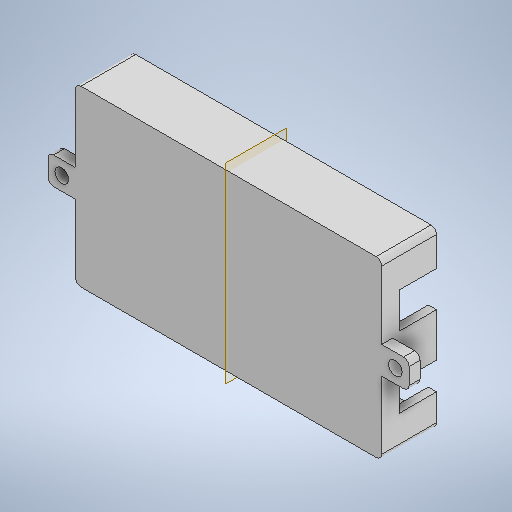
# Autodesk Inventor part: arduino_box
Saved by Autodesk Inventor 2025 (Build 290162000, 162)
## iProperties
Created: 2025-03-03
Part Number: arduino_box
Material: Všeobecné
Document SubType Name: Modeling
Designer: lukas
Density: 1 g/cm^3
Appearance: Výchozí
Author: lukas
## iProperties of the stored document arduino_box_3D tisk.ipt
Created: 2025-03-03
Part Number: arduino_box_3D tisk
Material: Všeobecné
Document SubType Name: Modeling
Designer: lukas
Density: 1 g/cm^3
Appearance: Výchozí
Author: lukas
Autodesk Inventor part; units mm, degrees
(part 1 of 2)
ref_plane "YZ Plane" through (0, 0, 0) normal (1, 0, 0) x (0, 1, 0)
ref_plane "XZ Plane" through (0, 0, 0) normal (0, 1, 0) x (-1, 0, 0)
sketch "Náčrt1" plane through (0, 0, 0) normal (0, 0, 1) x (1, 0, 0)
  line L0 (-99.06, 40.7162) -> (-101.6, 38.1762)
  line L1 (-101.6, 38.1762) -> (-101.6, 3.556)
  line L2 (-101.6, 3.556) -> (-98.044, 0)
  line L3 (-98.044, 0) -> (-1.524, 0)
  line L4 (-1.524, 0) -> (0, 1.524)
  line L5 (0, 1.524) -> (0, 51.8922)
  line L6 (0, 51.8922) -> (-1.524, 53.4162)
  line L7 (-1.524, 53.4162) -> (-97.2966, 53.4162)
  line L8 (-97.2966, 53.4162) -> (-99.06, 51.6528)
  line L9 (-99.06, 51.6528) -> (-99.06, 40.7162)
  circle A0 centre (-89.2556, 50.8762) radius 1.5621
  circle A1 centre (-65.7479, 35.4347) radius 1.3153
  circle A2 centre (-65.7479, 7.4185) radius 1.5621
  circle A3 centre (-96.7486, 2.54) radius 1.5621
  circle A4 centre (-14.1224, 2.54) radius 1.5621
  circle A5 centre (-14.1224, 50.8762) radius 1.5621
  line L10 (-91.7703, 3.1886) -> (-92.8414, 3.1886)
  line L11 (-91.7703, 1.1751) -> (-91.7703, 3.1886)
  line L12 (-92.8414, 1.1751) -> (-91.7703, 1.1751)
  line L13 (-92.8414, 3.1886) -> (-92.8414, 1.1751)
  line L14 (-86.6903, 1.1751) -> (-86.6903, 3.1886)
  line L15 (-87.7614, 1.1751) -> (-86.6903, 1.1751)
  line L16 (-87.7614, 3.1886) -> (-87.7614, 1.1751)
  line L17 (-86.6903, 3.1886) -> (-87.7614, 3.1886)
  line L18 (-81.6103, 1.1751) -> (-81.6103, 3.1886)
  line L19 (-82.6814, 1.1751) -> (-81.6103, 1.1751)
  line L20 (-82.6814, 3.1886) -> (-82.6814, 1.1751)
  line L21 (-81.6103, 3.1886) -> (-82.6814, 3.1886)
  line L22 (-76.5303, 1.1751) -> (-76.5303, 3.1886)
  line L23 (-77.6014, 1.1751) -> (-76.5303, 1.1751)
  line L24 (-77.6014, 3.1886) -> (-77.6014, 1.1751)
  line L25 (-76.5303, 3.1886) -> (-77.6014, 3.1886)
  line L26 (-68.6825, 3.4297) -> (-69.7244, 3.4297)
  line L27 (-68.6825, 1.346) -> (-68.6825, 3.4297)
  line L28 (-69.7244, 1.346) -> (-68.6825, 1.346)
  line L29 (-69.7244, 3.4297) -> (-69.7244, 1.346)
  line L30 (-63.6025, 1.346) -> (-63.6025, 3.4297)
  line L31 (-64.6444, 1.346) -> (-63.6025, 1.346)
  line L32 (-64.6444, 3.4297) -> (-64.6444, 1.346)
  line L33 (-63.6025, 3.4297) -> (-64.6444, 3.4297)
  line L34 (-58.5225, 1.346) -> (-58.5225, 3.4297)
  line L35 (-59.5644, 1.346) -> (-58.5225, 1.346)
  line L36 (-59.5644, 3.4297) -> (-59.5644, 1.346)
  line L37 (-58.5225, 3.4297) -> (-59.5644, 3.4297)
  line L38 (-53.4425, 1.346) -> (-53.4425, 3.4297)
  line L39 (-54.4844, 1.346) -> (-53.4425, 1.346)
  line L40 (-54.4844, 3.4297) -> (-54.4844, 1.346)
  line L41 (-53.4425, 3.4297) -> (-54.4844, 3.4297)
  line L42 (-45.4737, 3.6867) -> (-46.5774, 3.6867)
  line L43 (-45.4737, 1.6118) -> (-45.4737, 3.6867)
  line L44 (-46.5774, 1.6118) -> (-45.4737, 1.6118)
  line L45 (-46.5774, 3.6867) -> (-46.5774, 1.6118)
  line L46 (-40.3937, 1.6118) -> (-40.3937, 3.6867)
  line L47 (-41.4974, 1.6118) -> (-40.3937, 1.6118)
  line L48 (-41.4974, 3.6867) -> (-41.4974, 1.6118)
  line L49 (-40.3937, 3.6867) -> (-41.4974, 3.6867)
  line L50 (-35.3137, 1.6118) -> (-35.3137, 3.6867)
  line L51 (-36.4174, 1.6118) -> (-35.3137, 1.6118)
  line L52 (-36.4174, 3.6867) -> (-36.4174, 1.6118)
  line L53 (-35.3137, 3.6867) -> (-36.4174, 3.6867)
  circle A6 centre (-97.5648, 7.2848) radius 0.5739
  circle A7 centre (-95.0248, 7.2848) radius 0.5739
  circle A8 centre (-95.0248, 9.8248) radius 0.5739
  circle A9 centre (-95.0248, 12.3648) radius 0.5739
  circle A10 centre (-95.0248, 14.9048) radius 0.5739
  circle A11 centre (-95.0248, 17.4448) radius 0.5739
  circle A12 centre (-95.0248, 19.9848) radius 0.5739
  circle A13 centre (-95.0248, 22.5248) radius 0.5739
  circle A14 centre (-95.0248, 25.0648) radius 0.5739
  circle A15 centre (-95.0248, 27.6048) radius 0.5739
  circle A16 centre (-95.0248, 30.1448) radius 0.5739
  circle A17 centre (-95.0248, 32.6848) radius 0.5739
  circle A18 centre (-95.0248, 35.2248) radius 0.5739
  circle A19 centre (-95.0248, 37.7648) radius 0.5739
  circle A20 centre (-95.0248, 40.3048) radius 0.5739
  circle A21 centre (-95.0248, 42.8448) radius 0.5739
  circle A22 centre (-95.0248, 45.3848) radius 0.5739
  circle A23 centre (-95.0248, 47.9248) radius 0.5739
  circle A24 centre (-95.0248, 50.4648) radius 0.5739
  line L54 (-81.8933, 50.0717) -> (-81.8933, 51.6679)
  line L55 (-82.3984, 50.0717) -> (-81.8933, 50.0717)
  line L56 (-82.3984, 51.6679) -> (-82.3984, 50.0717)
  line L57 (-81.8933, 51.6679) -> (-82.3984, 51.6679)
  line L58 (-76.8133, 50.0717) -> (-76.8133, 51.6679)
  line L59 (-77.3184, 50.0717) -> (-76.8133, 50.0717)
  line L60 (-77.3184, 51.6679) -> (-77.3184, 50.0717)
  line L61 (-76.8133, 51.6679) -> (-77.3184, 51.6679)
  line L62 (-71.7333, 50.0717) -> (-71.7333, 51.6679)
  line L63 (-72.2384, 50.0717) -> (-71.7333, 50.0717)
  line L64 (-72.2384, 51.6679) -> (-72.2384, 50.0717)
  line L65 (-71.7333, 51.6679) -> (-72.2384, 51.6679)
  line L66 (-63.4227, 51.9137) -> (-64.2563, 51.9137)
  line L67 (-63.4227, 50.0717) -> (-63.4227, 51.9137)
  line L68 (-64.2563, 50.0717) -> (-63.4227, 50.0717)
  line L69 (-64.2563, 51.9137) -> (-64.2563, 50.0717)
  line L70 (-58.3427, 50.0717) -> (-58.3427, 51.9137)
  line L71 (-59.1763, 50.0717) -> (-58.3427, 50.0717)
  line L72 (-59.1763, 51.9137) -> (-59.1763, 50.0717)
  line L73 (-58.3427, 51.9137) -> (-59.1763, 51.9137)
  line L74 (-53.2627, 50.0717) -> (-53.2627, 51.9137)
  line L75 (-54.0963, 50.0717) -> (-53.2627, 50.0717)
  line L76 (-54.0963, 51.9137) -> (-54.0963, 50.0717)
  line L77 (-53.2627, 51.9137) -> (-54.0963, 51.9137)
  line L78 (-48.1827, 50.0717) -> (-48.1827, 51.9137)
  line L79 (-49.0163, 50.0717) -> (-48.1827, 50.0717)
  line L80 (-49.0163, 51.9137) -> (-49.0163, 50.0717)
  line L81 (-48.1827, 51.9137) -> (-49.0163, 51.9137)
  line L82 (-41.4974, 51.9137) -> (-42.4723, 51.9137)
  line L83 (-41.4974, 50.0717) -> (-41.4974, 51.9137)
  line L84 (-42.4723, 50.0717) -> (-41.4974, 50.0717)
  line L85 (-42.4723, 51.9137) -> (-42.4723, 50.0717)
  line L86 (-36.4174, 50.0717) -> (-36.4174, 51.9137)
  line L87 (-37.3923, 50.0717) -> (-36.4174, 50.0717)
  line L88 (-37.3923, 51.9137) -> (-37.3923, 50.0717)
  line L89 (-36.4174, 51.9137) -> (-37.3923, 51.9137)
  line L90 (-31.3374, 50.0717) -> (-31.3374, 51.9137)
  line L91 (-32.3123, 50.0717) -> (-31.3374, 50.0717)
  line L92 (-32.3123, 51.9137) -> (-32.3123, 50.0717)
  line L93 (-31.3374, 51.9137) -> (-32.3123, 51.9137)
  line L94 (-26.2574, 50.0717) -> (-26.2574, 51.9137)
  line L95 (-27.2323, 50.0717) -> (-26.2574, 50.0717)
  line L96 (-27.2323, 51.9137) -> (-27.2323, 50.0717)
  line L97 (-26.2574, 51.9137) -> (-27.2323, 51.9137)
  circle A25 centre (-20.5945, 47.6784) radius 0.5437
  circle A26 centre (-18.0545, 47.6784) radius 0.5437
  circle A27 centre (-20.5945, 45.1384) radius 0.5437
  circle A28 centre (-15.5145, 45.1384) radius 0.5437
  circle A29 centre (-5.7466, 39.5769) radius 0.4144
  circle A30 centre (-5.7466, 37.0369) radius 0.4144
  line L98 (-7.393, 4.043) -> (-10.0091, 4.043)
  line L99 (-7.393, 3.3305) -> (-7.393, 4.043)
  line L100 (-10.0091, 3.3305) -> (-7.393, 3.3305)
  line L101 (-10.0091, 4.043) -> (-10.0091, 3.3305)
  line L102 (-2.4767, 32.5537) -> (-4.2776, 32.5537)
  line L103 (-2.4767, 31.6979) -> (-2.4767, 32.5537)
  line L104 (-4.2776, 31.6979) -> (-2.4767, 31.6979)
  line L105 (-4.2776, 32.5537) -> (-4.2776, 31.6979)
  line L106 (-2.249, 44.6927) -> (-4.5054, 44.6927)
  line L107 (-2.249, 43.8153) -> (-2.249, 44.6927)
  line L108 (-4.5054, 43.8153) -> (-2.249, 43.8153)
  line L109 (-4.5054, 44.6927) -> (-4.5054, 43.8153)
  line L110 (-5.2737, 10.2292) -> (-5.7128, 10.2292)
  line L111 (-5.2737, 7.3652) -> (-5.2737, 10.2292)
  line L112 (-5.7128, 7.3652) -> (-5.2737, 7.3652)
  line L113 (-5.7128, 10.2292) -> (-5.7128, 7.3652)
  circle A31 centre (-8.2866, 37.0369) radius 0.4144
  line L114 (-11.4599, 10.2292) -> (-12.1472, 10.2292)
  line L115 (-11.4599, 7.3652) -> (-11.4599, 10.2292)
  line L116 (-12.1472, 7.3652) -> (-11.4599, 7.3652)
  line L117 (-12.1472, 10.2292) -> (-12.1472, 7.3652)
  circle A32 centre (-18.0545, 45.1384) radius 0.5437
  circle A33 centre (-15.5145, 47.6784) radius 0.5437
  circle A34 centre (-8.2866, 39.5769) radius 0.4144
  line L118 (-23.7174, 50.0717) -> (-23.7174, 51.9137)
  line L119 (-24.6923, 50.0717) -> (-23.7174, 50.0717)
  line L120 (-24.6923, 51.9137) -> (-24.6923, 50.0717)
  line L121 (-23.7174, 51.9137) -> (-24.6923, 51.9137)
  line L122 (-28.7974, 50.0717) -> (-28.7974, 51.9137)
  line L123 (-29.7723, 50.0717) -> (-28.7974, 50.0717)
  line L124 (-29.7723, 51.9137) -> (-29.7723, 50.0717)
  line L125 (-28.7974, 51.9137) -> (-29.7723, 51.9137)
  line L126 (-33.8774, 50.0717) -> (-33.8774, 51.9137)
  line L127 (-34.8523, 50.0717) -> (-33.8774, 50.0717)
  line L128 (-34.8523, 51.9137) -> (-34.8523, 50.0717)
  line L129 (-33.8774, 51.9137) -> (-34.8523, 51.9137)
  line L130 (-38.9574, 50.0717) -> (-38.9574, 51.9137)
  line L131 (-39.9323, 50.0717) -> (-38.9574, 50.0717)
  line L132 (-39.9323, 51.9137) -> (-39.9323, 50.0717)
  line L133 (-38.9574, 51.9137) -> (-39.9323, 51.9137)
  line L134 (-45.6427, 50.0717) -> (-45.6427, 51.9137)
  line L135 (-46.4763, 50.0717) -> (-45.6427, 50.0717)
  line L136 (-46.4763, 51.9137) -> (-46.4763, 50.0717)
  line L137 (-45.6427, 51.9137) -> (-46.4763, 51.9137)
  line L138 (-50.7227, 50.0717) -> (-50.7227, 51.9137)
  line L139 (-51.5563, 50.0717) -> (-50.7227, 50.0717)
  line L140 (-51.5563, 51.9137) -> (-51.5563, 50.0717)
  line L141 (-50.7227, 51.9137) -> (-51.5563, 51.9137)
  line L142 (-55.8027, 50.0717) -> (-55.8027, 51.9137)
  line L143 (-56.6363, 50.0717) -> (-55.8027, 50.0717)
  line L144 (-56.6363, 51.9137) -> (-56.6363, 50.0717)
  line L145 (-55.8027, 51.9137) -> (-56.6363, 51.9137)
  line L146 (-60.8827, 50.0717) -> (-60.8827, 51.9137)
  line L147 (-61.7163, 50.0717) -> (-60.8827, 50.0717)
  line L148 (-61.7163, 51.9137) -> (-61.7163, 50.0717)
  line L149 (-60.8827, 51.9137) -> (-61.7163, 51.9137)
  line L150 (-69.1933, 50.0717) -> (-69.1933, 51.6679)
  line L151 (-69.6984, 50.0717) -> (-69.1933, 50.0717)
  line L152 (-69.6984, 51.6679) -> (-69.6984, 50.0717)
  line L153 (-69.1933, 51.6679) -> (-69.6984, 51.6679)
  line L154 (-74.2733, 50.0717) -> (-74.2733, 51.6679)
  line L155 (-74.7784, 50.0717) -> (-74.2733, 50.0717)
  line L156 (-74.7784, 51.6679) -> (-74.7784, 50.0717)
  line L157 (-74.2733, 51.6679) -> (-74.7784, 51.6679)
  line L158 (-79.3533, 50.0717) -> (-79.3533, 51.6679)
  line L159 (-79.8584, 50.0717) -> (-79.3533, 50.0717)
  line L160 (-79.8584, 51.6679) -> (-79.8584, 50.0717)
  line L161 (-79.3533, 51.6679) -> (-79.8584, 51.6679)
  line L162 (-84.4333, 50.0717) -> (-84.4333, 51.6679)
  line L163 (-84.9384, 50.0717) -> (-84.4333, 50.0717)
  line L164 (-84.9384, 51.6679) -> (-84.9384, 50.0717)
  line L165 (-84.4333, 51.6679) -> (-84.9384, 51.6679)
  circle A35 centre (-97.5648, 50.4648) radius 0.5739
  circle A36 centre (-97.5648, 47.9248) radius 0.5739
  circle A37 centre (-97.5648, 45.3848) radius 0.5739
  circle A38 centre (-97.5648, 42.8448) radius 0.5739
  circle A39 centre (-97.5648, 40.3048) radius 0.5739
  circle A40 centre (-97.5648, 37.7648) radius 0.5739
  circle A41 centre (-97.5648, 35.2248) radius 0.5739
  circle A42 centre (-97.5648, 32.6848) radius 0.5739
  circle A43 centre (-97.5648, 30.1448) radius 0.5739
  circle A44 centre (-97.5648, 27.6048) radius 0.5739
  circle A45 centre (-97.5648, 25.0648) radius 0.5739
  circle A46 centre (-97.5648, 22.5248) radius 0.5739
  circle A47 centre (-97.5648, 19.9848) radius 0.5739
  circle A48 centre (-97.5648, 17.4448) radius 0.5739
  circle A49 centre (-97.5648, 14.9048) radius 0.5739
  circle A50 centre (-97.5648, 12.3648) radius 0.5739
  circle A51 centre (-97.5648, 9.8248) radius 0.5739
  line L166 (-86.9733, 51.6679) -> (-87.4784, 51.6679)
  line L167 (-86.9733, 50.0717) -> (-86.9733, 51.6679)
  line L168 (-87.4784, 50.0717) -> (-86.9733, 50.0717)
  line L169 (-87.4784, 51.6679) -> (-87.4784, 50.0717)
  line L170 (-32.7737, 1.6118) -> (-32.7737, 3.6867)
  line L171 (-33.8774, 1.6118) -> (-32.7737, 1.6118)
  line L172 (-33.8774, 3.6867) -> (-33.8774, 1.6118)
  line L173 (-32.7737, 3.6867) -> (-33.8774, 3.6867)
  line L174 (-37.8537, 1.6118) -> (-37.8537, 3.6867)
  line L175 (-38.9574, 1.6118) -> (-37.8537, 1.6118)
  line L176 (-38.9574, 3.6867) -> (-38.9574, 1.6118)
  line L177 (-37.8537, 3.6867) -> (-38.9574, 3.6867)
  line L178 (-42.9337, 1.6118) -> (-42.9337, 3.6867)
  line L179 (-44.0374, 1.6118) -> (-42.9337, 1.6118)
  line L180 (-44.0374, 3.6867) -> (-44.0374, 1.6118)
  line L181 (-42.9337, 3.6867) -> (-44.0374, 3.6867)
  line L182 (-50.9025, 1.346) -> (-50.9025, 3.4297)
  line L183 (-51.9444, 1.346) -> (-50.9025, 1.346)
  line L184 (-51.9444, 3.4297) -> (-51.9444, 1.346)
  line L185 (-50.9025, 3.4297) -> (-51.9444, 3.4297)
  line L186 (-55.9825, 1.346) -> (-55.9825, 3.4297)
  line L187 (-57.0244, 1.346) -> (-55.9825, 1.346)
  line L188 (-57.0244, 3.4297) -> (-57.0244, 1.346)
  line L189 (-55.9825, 3.4297) -> (-57.0244, 3.4297)
  line L190 (-61.0625, 1.346) -> (-61.0625, 3.4297)
  line L191 (-62.1044, 1.346) -> (-61.0625, 1.346)
  line L192 (-62.1044, 3.4297) -> (-62.1044, 1.346)
  line L193 (-61.0625, 3.4297) -> (-62.1044, 3.4297)
  line L194 (-66.1425, 1.346) -> (-66.1425, 3.4297)
  line L195 (-67.1844, 1.346) -> (-66.1425, 1.346)
  line L196 (-67.1844, 3.4297) -> (-67.1844, 1.346)
  line L197 (-66.1425, 3.4297) -> (-67.1844, 3.4297)
  line L198 (-73.9903, 1.1751) -> (-73.9903, 3.1886)
  line L199 (-75.0614, 1.1751) -> (-73.9903, 1.1751)
  line L200 (-75.0614, 3.1886) -> (-75.0614, 1.1751)
  line L201 (-73.9903, 3.1886) -> (-75.0614, 3.1886)
  line L202 (-79.0703, 1.1751) -> (-79.0703, 3.1886)
  line L203 (-80.1414, 1.1751) -> (-79.0703, 1.1751)
  line L204 (-80.1414, 3.1886) -> (-80.1414, 1.1751)
  line L205 (-79.0703, 3.1886) -> (-80.1414, 3.1886)
  line L206 (-84.1503, 1.1751) -> (-84.1503, 3.1886)
  line L207 (-85.2214, 1.1751) -> (-84.1503, 1.1751)
  line L208 (-85.2214, 3.1886) -> (-85.2214, 1.1751)
  line L209 (-84.1503, 3.1886) -> (-85.2214, 3.1886)
  line L210 (-89.2303, 1.1751) -> (-89.2303, 3.1886)
  line L211 (-90.3014, 1.1751) -> (-89.2303, 1.1751)
  line L212 (-90.3014, 3.1886) -> (-90.3014, 1.1751)
  line L213 (-89.2303, 3.1886) -> (-90.3014, 3.1886)
  line L214 (0, 64.0994) -> (0, -10.6832)
  line L215 (-121.92, 0) -> (20.32, 0)
  line L216 (0, 0) -> (-101.6, 0)
  line L217 (-101.6, 0) -> (-101.6, 53.4162)
  line L218 (-101.6, 53.4162) -> (0, 53.4162)
  line L219 (0, 53.4162) -> (0, 0)
  dimension "d0" = 0
  constraints: 8 end point, 2 parallel, 1 horizontal, 1 perpendicular, 1 point on line
  measures "d0" distance between parallel lines of L1 L217
extrude "Vysunutí1" add sketch "Náčrt1" along normal blind 2 contours L9 L8 L7 L6 L5 L4 L3 L2 L1 L0 | L0 L217 L218 L8 L9 | L2 L215 L217 | L218 L214 L6 | L4 L214 L215 | A0 | A1 | A2 | A3 | A4 | A5 | L11 L12 L13 L10 | L15 L16 L17 L14 | L19 L20 L21 L18 | L23 L24 L25 L22 | L27 L28 L29 L26 | L31 L32 L33 L30 | L35 L36 L37 L34 | L39 L40 L41 L38 | L43 L44 L45 L42 | L47 L48 L49 L46 | L51 L52 L53 L50 | A6 | A7 | A8 | A9 | A10 | A11 | A12 | A13 | A14 | A15 | A16 | A17 | A18 | A19 | A20 | A21 | A22 | A23 | A24 | L55 L56 L57 L54 | L59 L60 L61 L58 | L63 L64 L65 L62 | L67 L68 L69 L66 | L71 L72 L73 L70 | L75 L76 L77 L74 | L79 L80 L81 L78 | L83 L84 L85 L82 | L87 L88 L89 L86 | L91 L92 L93 L90 | L95 L96 L97 L94 | A25 | A26 | A27 | A28 | A29 | A30 | L99 L100 L101 L98 | L103 L104 L105 L102 | L107 L108 L109 L106 | L111 L112 L113 L110 | A31 | L115 L116 L117 L114 | A32 | A33 | A34 | L119 L120 L121 L118 | L123 L124 L125 L122 | L127 L128 L129 L126 | L131 L132 L133 L130 | L135 L136 L137 L134 | L139 L140 L141 L138 | L143 L144 L145 L142 | L147 L148 L149 L146 | L151 L152 L153 L150 | L155 L156 L157 L154 | L159 L160 L161 L158 | L163 L164 L165 L162 | A35 | A36 | A37 | A38 | A39 | A40 | A41 | A42 | A43 | A44 | A45 | A46 | A47 | A48 | A49 | A50 | A51 | L167 L168 L169 L166 | L171 L172 L173 L170 | L175 L176 L177 L174 | L179 L180 L181 L178 | L183 L184 L185 L182 | L187 L188 L189 L186 | L191 L192 L193 L190 | L195 L196 L197 L194 | L199 L200 L201 L198 | L203 L204 L205 L202 | L207 L208 L209 L206 | L211 L212 L213 L210
sketch "Náčrt2" plane through (0, 0, 0) normal (0, 0, -1) x (-1, 0, 0)
  line L0 (10.795, 12.8905) -> (10.795, 12.2555)
  arc A0 (10.795, 12.2555) -> (10.8585, 12.192) centre (10.8585, 12.2555) ccw
  line L1 (10.8585, 12.192) -> (12.3317, 12.192)
  arc A1 (12.3952, 12.1285) -> (12.3317, 12.192) centre (12.3317, 12.1285) ccw
  line L2 (12.3952, 4.6355) -> (12.3952, 12.1285)
  arc A2 (12.3317, 4.572) -> (12.3952, 4.6355) centre (12.3317, 4.6355) ccw
  line L3 (12.3317, 4.572) -> (10.8585, 4.572)
  arc A3 (10.8585, 4.572) -> (10.795, 4.5085) centre (10.8585, 4.5085) ccw
  line L4 (10.795, 4.5085) -> (10.795, 3.8735)
  arc A4 (10.7315, 3.81) -> (10.795, 3.8735) centre (10.7315, 3.8735) ccw
  line L5 (0, 3.81) -> (10.7315, 3.81)
  line L6 (0, 1.524) -> (0, 3.81)
  line L7 (0, 1.524) -> (1.524, 0)
  line L8 (98.044, 0) -> (1.524, 0)
  line L9 (98.044, 0) -> (101.6, 3.556)
  line L10 (101.6, 38.1762) -> (101.6, 3.556)
  line L11 (99.06, 40.7162) -> (101.6, 38.1762)
  line L12 (99.06, 51.6528) -> (99.06, 40.7162)
  line L13 (97.2966, 53.4162) -> (99.06, 51.6528)
  line L14 (1.524, 53.4162) -> (97.2966, 53.4162)
  line L15 (1.524, 53.4162) -> (0, 51.8922)
  line L16 (0, 44.1452) -> (0, 51.8922)
  line L17 (7.0104, 44.1452) -> (0, 44.1452)
  line L18 (7.0104, 44.2087) -> (7.0104, 44.1452)
  line L19 (9.9568, 44.2087) -> (7.0104, 44.2087)
  line L20 (9.9568, 32.1437) -> (9.9568, 44.2087)
  line L21 (9.9568, 32.1437) -> (7.0104, 32.1437)
  line L22 (7.0104, 32.1437) -> (7.0104, 32.2072)
  line L23 (0, 32.2072) -> (7.0104, 32.2072)
  line L24 (0, 12.954) -> (0, 32.2072)
  line L25 (10.7315, 12.954) -> (0, 12.954)
  arc A5 (10.795, 12.8905) -> (10.7315, 12.954) centre (10.7315, 12.8905) ccw
  line L26 (47.625, 1.3462) -> (47.625, 3.7956)
  line L27 (31.9278, 1.3462) -> (47.625, 1.3462)
  line L28 (31.9278, 3.7956) -> (31.9278, 1.3462)
  line L29 (47.625, 3.7956) -> (31.9278, 3.7956)
  line L30 (21.2598, 49.6824) -> (42.0116, 49.6824)
  line L31 (21.2598, 52.1462) -> (21.2598, 49.6824)
  line L32 (42.0116, 52.1462) -> (21.2598, 52.1462)
  line L33 (42.0116, 49.6824) -> (42.0116, 52.1462)
  line L34 (72.517, 3.81) -> (72.517, 1.3462)
  line L35 (93.345, 3.81) -> (72.517, 3.81)
  line L36 (93.345, 1.3462) -> (93.345, 3.81)
  line L37 (72.517, 1.3462) -> (93.345, 1.3462)
  line L38 (97.536, 5.9182) -> (97.536, 52.197)
  line L39 (92.5576, 5.9182) -> (97.536, 5.9182)
  line L40 (92.5576, 52.197) -> (92.5576, 5.9182)
  line L41 (97.536, 52.197) -> (92.5576, 52.197)
  line L42 (66.7258, 52.1462) -> (66.7258, 49.6824)
  line L43 (87.4776, 52.1462) -> (66.7258, 52.1462)
  line L44 (87.4776, 49.6824) -> (87.4776, 52.1462)
  line L45 (66.7258, 49.6824) -> (87.4776, 49.6824)
  line L46 (43.9928, 49.6824) -> (64.7446, 49.6824)
  line L47 (43.9928, 52.1462) -> (43.9928, 49.6824)
  line L48 (64.7446, 52.1462) -> (43.9928, 52.1462)
  line L49 (64.7446, 49.6824) -> (64.7446, 52.1462)
  line L50 (49.784, 1.3462) -> (70.612, 1.3462)
  line L51 (49.784, 3.81) -> (49.784, 1.3462)
  line L52 (70.612, 3.81) -> (49.784, 3.81)
  line L53 (70.612, 1.3462) -> (70.612, 3.81)
  line L54 (26.4691, 25.5422) -> (26.4691, 24.1341)
  line L55 (29.2341, 25.5422) -> (26.4691, 25.5422)
  line L56 (29.2341, 24.1341) -> (29.2341, 25.5422)
  line L57 (26.4691, 24.1341) -> (29.2341, 24.1341)
  line L58 (6.8597, 20.6667) -> (6.8597, 14.174)
  line L59 (10.1287, 20.6667) -> (6.8597, 20.6667)
  line L60 (10.1287, 14.174) -> (10.1287, 20.6667)
  line L61 (6.8597, 14.174) -> (10.1287, 14.174)
  line L62 (17.0001, 22.4519) -> (17.0001, 19.5908)
  line L63 (19.8206, 22.4519) -> (17.0001, 22.4519)
  line L64 (19.8206, 19.5908) -> (19.8206, 22.4519)
  line L65 (17.0001, 19.5908) -> (19.8206, 19.5908)
  line L66 (20.7541, 17.2167) -> (20.7541, 16.4862)
  line L67 (22.3503, 17.2167) -> (20.7541, 17.2167)
  line L68 (22.3503, 16.4862) -> (22.3503, 17.2167)
  line L69 (20.7541, 16.4862) -> (22.3503, 16.4862)
  line L70 (2.6828, 28.6543) -> (2.6828, 24.1341)
  line L71 (5.8459, 28.6543) -> (2.6828, 28.6543)
  line L72 (5.8459, 24.1341) -> (5.8459, 28.6543)
  line L73 (2.6828, 24.1341) -> (5.8459, 24.1341)
  line L74 (37.9203, 7.1822) -> (37.9203, 6.4561)
  line L75 (39.468, 7.1822) -> (37.9203, 7.1822)
  line L76 (39.468, 6.4561) -> (39.468, 7.1822)
  line L77 (37.9203, 6.4561) -> (39.468, 6.4561)
  line L78 (40.0898, 15.0906) -> (40.0898, 13.6337)
  line L79 (41.0914, 15.0906) -> (40.0898, 15.0906)
  line L80 (41.0914, 13.6337) -> (41.0914, 15.0906)
  line L81 (40.0898, 13.6337) -> (41.0914, 13.6337)
  line L82 (34.709, 15.9464) -> (34.709, 12.6868)
  line L83 (36.5608, 15.9464) -> (34.709, 15.9464)
  line L84 (36.5608, 12.6868) -> (36.5608, 15.9464)
  line L85 (34.709, 12.6868) -> (36.5608, 12.6868)
  line L86 (27.2293, 21.6382) -> (27.2293, 20.877)
  line L87 (28.7931, 21.6382) -> (27.2293, 21.6382)
  line L88 (28.7931, 20.877) -> (28.7931, 21.6382)
  line L89 (27.2293, 20.877) -> (28.7931, 20.877)
  line L90 (11.2848, 29.3883) -> (11.2848, 28.6543)
  line L91 (12.7546, 29.3883) -> (11.2848, 29.3883)
  line L92 (12.7546, 28.6543) -> (12.7546, 29.3883)
  line L93 (11.2848, 28.6543) -> (12.7546, 28.6543)
  line L94 (17.6277, 29.5208) -> (17.6277, 28.6543)
  line L95 (19.2035, 29.5208) -> (17.6277, 29.5208)
  line L96 (19.2035, 28.6543) -> (19.2035, 29.5208)
  line L97 (17.6277, 28.6543) -> (19.2035, 28.6543)
  line L98 (23.859, 29.5208) -> (23.859, 28.6543)
  line L99 (25.4224, 29.5208) -> (23.859, 29.5208)
  line L100 (25.4224, 28.6543) -> (25.4224, 29.5208)
  line L101 (23.859, 28.6543) -> (25.4224, 28.6543)
  line L102 (26.9146, 34.715) -> (26.9146, 33.4422)
  line L103 (28.6926, 34.715) -> (26.9146, 34.715)
  line L104 (28.6926, 33.4422) -> (28.6926, 34.715)
  line L105 (26.9146, 33.4422) -> (28.6926, 33.4422)
  line L106 (27.4303, 40.8048) -> (27.4303, 37.5488)
  line L107 (28.2839, 40.8048) -> (27.4303, 40.8048)
  line L108 (28.2839, 37.5488) -> (28.2839, 40.8048)
  line L109 (27.4303, 37.5488) -> (28.2839, 37.5488)
  line L110 (27.0516, 44.6498) -> (27.0516, 43.8951)
  line L111 (28.4879, 44.6498) -> (27.0516, 44.6498)
  line L112 (28.4879, 43.8951) -> (28.4879, 44.6498)
  line L113 (27.0516, 43.8951) -> (28.4879, 43.8951)
  line L114 (11.1523, 42.3897) -> (11.1523, 41.6172)
  line L115 (12.7546, 42.3897) -> (11.1523, 42.3897)
  line L116 (12.7546, 41.6172) -> (12.7546, 42.3897)
  line L117 (11.1523, 41.6172) -> (12.7546, 41.6172)
  line L118 (11.4503, 38.4446) -> (11.4503, 35.2712)
  line L119 (12.4133, 38.4446) -> (11.4503, 38.4446)
  line L120 (12.4133, 35.2712) -> (12.4133, 38.4446)
  line L121 (11.4503, 35.2712) -> (12.4133, 35.2712)
  line L122 (75.6756, 37.5488) -> (75.6756, 36.1287)
  line L123 (77.4802, 37.5488) -> (75.6756, 37.5488)
  line L124 (77.4802, 36.1287) -> (77.4802, 37.5488)
  line L125 (75.6756, 36.1287) -> (77.4802, 36.1287)
  line L126 (11.8224, 47.7016) -> (11.8224, 44.4497)
  line L127 (13.6426, 47.7016) -> (11.8224, 47.7016)
  line L128 (13.6426, 44.4497) -> (13.6426, 47.7016)
  line L129 (11.8224, 44.4497) -> (13.6426, 44.4497)
  arc A6 (14.5172, 27.5532) -> (14.5172, 23.7943) centre (14.8394, 25.6738) ccw
  line L130 (22.4159, 27.5532) -> (14.5172, 27.5532)
  arc A7 (22.4159, 23.7943) -> (22.4159, 27.5532) centre (22.0937, 25.6738) ccw
  line L131 (14.5172, 23.7943) -> (22.4159, 23.7943)
  circle A8 centre (25.2188, 8.6007) radius 3.302
  line L132 (67.919, 27.2067) -> (67.919, 27.8713)
  line L133 (66.903, 26.1907) -> (67.919, 27.2067)
  line L134 (63.5244, 26.1907) -> (66.903, 26.1907)
  line L135 (62.5084, 27.2067) -> (63.5244, 26.1907)
  line L136 (62.5084, 27.8713) -> (62.5084, 27.2067)
  line L137 (63.5244, 28.8873) -> (62.5084, 27.8713)
  line L138 (66.903, 28.8873) -> (63.5244, 28.8873)
  line L139 (67.919, 27.8713) -> (66.903, 28.8873)
  line L140 (15.9051, 48.775) -> (15.2447, 48.775)
  line L141 (16.9211, 47.759) -> (15.9051, 48.775)
  line L142 (16.9211, 44.3808) -> (16.9211, 47.759)
  line L143 (15.9051, 43.3648) -> (16.9211, 44.3808)
  line L144 (15.2447, 43.3648) -> (15.9051, 43.3648)
  line L145 (14.2287, 44.3808) -> (15.2447, 43.3648)
  line L146 (14.2287, 47.759) -> (14.2287, 44.3808)
  line L147 (15.2447, 48.775) -> (14.2287, 47.759)
  line L148 (20.8327, 48.775) -> (19.8167, 47.759)
  line L149 (21.4931, 48.775) -> (20.8327, 48.775)
  line L150 (22.5091, 47.759) -> (21.4931, 48.775)
  line L151 (22.5091, 44.3808) -> (22.5091, 47.759)
  line L152 (21.4931, 43.3648) -> (22.5091, 44.3808)
  line L153 (20.8327, 43.3648) -> (21.4931, 43.3648)
  line L154 (19.8167, 44.3808) -> (20.8327, 43.3648)
  line L155 (19.8167, 47.759) -> (19.8167, 44.3808)
  circle A9 centre (14.1224, 50.8762) radius 1.5621
  circle A10 centre (14.1224, 2.54) radius 1.5621
  circle A11 centre (96.7486, 2.54) radius 1.5621
  circle A12 centre (65.7479, 7.4185) radius 1.5621
  circle A13 centre (65.7479, 35.4347) radius 1.3153
  circle A14 centre (89.2556, 50.8762) radius 1.5621
  line L156 (18.0387, 48.775) -> (17.0227, 47.759)
  line L157 (18.6991, 48.775) -> (18.0387, 48.775)
  line L158 (19.7151, 47.759) -> (18.6991, 48.775)
  line L159 (19.7151, 44.3808) -> (19.7151, 47.759)
  line L160 (18.6991, 43.3648) -> (19.7151, 44.3808)
  line L161 (18.0387, 43.3648) -> (18.6991, 43.3648)
  line L162 (17.0227, 44.3808) -> (18.0387, 43.3648)
  line L163 (17.0227, 47.759) -> (17.0227, 44.3808)
  line L164 (67.919, 24.4127) -> (67.919, 25.0773)
  line L165 (66.903, 23.3967) -> (67.919, 24.4127)
  line L166 (63.5244, 23.3967) -> (66.903, 23.3967)
  line L167 (62.5084, 24.4127) -> (63.5244, 23.3967)
  line L168 (62.5084, 25.0773) -> (62.5084, 24.4127)
  line L169 (63.5244, 26.0933) -> (62.5084, 25.0773)
  line L170 (66.903, 26.0933) -> (63.5244, 26.0933)
  line L171 (67.919, 25.0773) -> (66.903, 26.0933)
  line L172 (67.919, 30.0007) -> (67.919, 30.6653)
  line L173 (66.903, 28.9847) -> (67.919, 30.0007)
  line L174 (63.5244, 28.9847) -> (66.903, 28.9847)
  line L175 (62.5084, 30.0007) -> (63.5244, 28.9847)
  line L176 (62.5084, 30.6653) -> (62.5084, 30.0007)
  line L177 (63.5244, 31.6813) -> (62.5084, 30.6653)
  line L178 (66.903, 31.6813) -> (63.5244, 31.6813)
  line L179 (67.919, 30.6653) -> (66.903, 31.6813)
  circle A15 centre (18.0299, 8.6007) radius 3.302
  line L180 (71.3142, 30.7771) -> (71.3142, 24.4981)
  line L181 (77.7751, 30.7771) -> (71.3142, 30.7771)
  line L182 (77.7751, 24.4981) -> (77.7751, 30.7771)
  line L183 (71.3142, 24.4981) -> (77.7751, 24.4981)
  line L184 (80.4259, 38.4446) -> (80.4259, 35.0406)
  line L185 (81.6732, 38.4446) -> (80.4259, 38.4446)
  line L186 (81.6732, 35.0406) -> (81.6732, 38.4446)
  line L187 (80.4259, 35.0406) -> (81.6732, 35.0406)
  line L188 (11.1523, 34.5656) -> (11.1523, 33.6296)
  line L189 (12.7546, 34.5656) -> (11.1523, 34.5656)
  line L190 (12.7546, 33.6296) -> (12.7546, 34.5656)
  line L191 (11.1523, 33.6296) -> (12.7546, 33.6296)
  line L192 (11.1523, 40.0722) -> (11.1523, 39.1768)
  line L193 (12.7546, 40.0722) -> (11.1523, 40.0722)
  line L194 (12.7546, 39.1768) -> (12.7546, 40.0722)
  line L195 (11.1523, 39.1768) -> (12.7546, 39.1768)
  line L196 (7.126, 45.5392) -> (7.126, 44.4497)
  line L197 (9.0679, 45.5392) -> (7.126, 45.5392)
  line L198 (9.0679, 44.4497) -> (9.0679, 45.5392)
  line L199 (7.126, 44.4497) -> (9.0679, 44.4497)
  line L200 (26.9146, 42.5941) -> (26.9146, 41.3621)
  line L201 (28.6926, 42.5941) -> (26.9146, 42.5941)
  line L202 (28.6926, 41.3621) -> (28.6926, 42.5941)
  line L203 (26.9146, 41.3621) -> (28.6926, 41.3621)
  line L204 (26.9146, 37.0281) -> (26.9146, 35.7687)
  line L205 (28.6926, 37.0281) -> (26.9146, 37.0281)
  line L206 (28.6926, 35.7687) -> (28.6926, 37.0281)
  line L207 (26.9146, 35.7687) -> (28.6926, 35.7687)
  line L208 (27.4303, 32.4686) -> (27.4303, 29.2498)
  line L209 (28.4879, 32.4686) -> (27.4303, 32.4686)
  line L210 (28.4879, 29.2498) -> (28.4879, 32.4686)
  line L211 (27.4303, 29.2498) -> (28.4879, 29.2498)
  line L212 (20.7541, 29.5208) -> (20.7541, 28.6543)
  line L213 (22.2343, 29.5208) -> (20.7541, 29.5208)
  line L214 (22.2343, 28.6543) -> (22.2343, 29.5208)
  line L215 (20.7541, 28.6543) -> (22.2343, 28.6543)
  line L216 (14.4129, 29.3883) -> (14.4129, 28.6543)
  line L217 (15.946, 29.3883) -> (14.4129, 29.3883)
  line L218 (15.946, 28.6543) -> (15.946, 29.3883)
  line L219 (14.4129, 28.6543) -> (15.946, 28.6543)
  line L220 (11.1523, 31.0171) -> (11.1523, 30.3418)
  line L221 (12.7546, 31.0171) -> (11.1523, 31.0171)
  line L222 (12.7546, 30.3418) -> (12.7546, 31.0171)
  line L223 (11.1523, 30.3418) -> (12.7546, 30.3418)
  line L224 (27.1372, 18.3326) -> (27.1372, 17.5844)
  line L225 (28.6926, 18.3326) -> (27.1372, 18.3326)
  line L226 (28.6926, 17.5844) -> (28.6926, 18.3326)
  line L227 (27.1372, 17.5844) -> (28.6926, 17.5844)
  line L228 (37.7953, 15.9464) -> (37.7953, 12.6868)
  line L229 (39.07, 15.9464) -> (37.7953, 15.9464)
  line L230 (39.07, 12.6868) -> (39.07, 15.9464)
  line L231 (37.7953, 12.6868) -> (39.07, 12.6868)
  line L232 (33.0606, 15.564) -> (33.0606, 13.4334)
  line L233 (34.0257, 15.564) -> (33.0606, 15.564)
  line L234 (34.0257, 13.4334) -> (34.0257, 15.564)
  line L235 (33.0606, 13.4334) -> (34.0257, 13.4334)
  line L236 (8.4942, 26.9002) -> (8.4942, 24.1341)
  line L237 (9.6416, 26.9002) -> (8.4942, 26.9002)
  line L238 (9.6416, 24.1341) -> (9.6416, 26.9002)
  line L239 (8.4942, 24.1341) -> (9.6416, 24.1341)
  line L240 (14.0173, 18.0486) -> (14.0173, 16.4862)
  line L241 (14.8086, 18.0486) -> (14.0173, 18.0486)
  line L242 (14.8086, 16.4862) -> (14.8086, 18.0486)
  line L243 (14.0173, 16.4862) -> (14.8086, 16.4862)
  line L244 (17.9944, 17.7848) -> (17.9944, 14.5787)
  line L245 (18.9481, 17.7848) -> (17.9944, 17.7848)
  line L246 (18.9481, 14.5787) -> (18.9481, 17.7848)
  line L247 (17.9944, 14.5787) -> (18.9481, 14.5787)
  line L248 (19.627, 3.6625) -> (19.627, 1.2157)
  line L249 (23.662, 3.6625) -> (19.627, 3.6625)
  line L250 (23.662, 1.2157) -> (23.662, 3.6625)
  line L251 (19.627, 1.2157) -> (23.662, 1.2157)
  line L252 (17.2908, 37.0281) -> (17.2908, 32.103)
  line L253 (22.3503, 37.0281) -> (17.2908, 37.0281)
  line L254 (22.3503, 32.103) -> (22.3503, 37.0281)
  line L255 (17.2908, 32.103) -> (22.3503, 32.103)
  line L256 (43.8395, 35.2712) -> (43.8395, 21.0732)
  line L257 (57.873, 35.2712) -> (43.8395, 35.2712)
  line L258 (57.873, 21.0732) -> (57.873, 35.2712)
  line L259 (43.8395, 21.0732) -> (57.873, 21.0732)
  circle A16 centre (96.7486, 2.54) radius 2.5
  circle A17 centre (89.2556, 50.8762) radius 2.5
  circle A18 centre (65.7479, 7.4185) radius 2.5
  circle A19 centre (65.7479, 35.4347) radius 2.5
  circle A20 centre (14.1224, 2.54) radius 2.5
  circle A21 centre (14.1224, 50.8762) radius 2.5
  point P0 (0, 0)
  dimension "d3" = 5
  dimension "d4" = 5
  dimension "d5" = 5
  dimension "d6" = 5
  dimension "d7" = 5
  dimension "d8" = 5
  constraints: 6 centre point, 6 coincident
  measures "d3" diameter of A16
  measures "d4" diameter of A17
  measures "d5" diameter of A18
  measures "d6" diameter of A19
  measures "d7" diameter of A20
  measures "d8" diameter of A21
extrude "Vysunutí2" add sketch "Náčrt2" along normal blind 2 contours A17 L45 L44 L43 | L43 L44 L45 A17 | A21 L147 L140 | L140 L147 A21 | A9 | A10 | A11 | A12 | A13 | A14 | A16 | A18 | A19 | A20
sketch "Náčrt3" plane through (-14.1224, 2.54, -2) normal (0, 0, -1) x (-1, 0, 0)
  line L0 (-3.3274, 10.3505) -> (-3.3274, 9.7155)
  arc A0 (-3.3274, 9.7155) -> (-3.2639, 9.652) centre (-3.2639, 9.7155) ccw
  line L1 (-3.2639, 9.652) -> (-1.7907, 9.652)
  arc A1 (-1.7272, 9.5885) -> (-1.7907, 9.652) centre (-1.7907, 9.5885) ccw
  line L2 (-1.7272, 2.0955) -> (-1.7272, 9.5885)
  arc A2 (-1.7907, 2.032) -> (-1.7272, 2.0955) centre (-1.7907, 2.0955) ccw
  line L3 (-1.7907, 2.032) -> (-3.2639, 2.032)
  arc A3 (-3.2639, 2.032) -> (-3.3274, 1.9685) centre (-3.2639, 1.9685) ccw
  line L4 (-3.3274, 1.9685) -> (-3.3274, 1.3335)
  arc A4 (-3.3909, 1.27) -> (-3.3274, 1.3335) centre (-3.3909, 1.3335) ccw
  line L5 (-14.1224, 1.27) -> (-3.3909, 1.27)
  line L6 (-14.1224, -1.016) -> (-14.1224, 1.27)
  line L7 (-14.1224, -1.016) -> (-12.5984, -2.54)
  line L8 (83.9216, -2.54) -> (-12.5984, -2.54)
  line L9 (83.9216, -2.54) -> (87.4776, 1.016)
  line L10 (87.4776, 35.6362) -> (87.4776, 1.016)
  line L11 (84.9376, 38.1762) -> (87.4776, 35.6362)
  line L12 (84.9376, 49.1128) -> (84.9376, 38.1762)
  line L13 (83.1742, 50.8762) -> (84.9376, 49.1128)
  line L14 (-12.5984, 50.8762) -> (83.1742, 50.8762)
  line L15 (-12.5984, 50.8762) -> (-14.1224, 49.3522)
  line L16 (-14.1224, 41.6052) -> (-14.1224, 49.3522)
  line L17 (-7.112, 41.6052) -> (-14.1224, 41.6052)
  line L18 (-7.112, 41.6687) -> (-7.112, 41.6052)
  line L19 (-4.1656, 41.6687) -> (-7.112, 41.6687)
  line L20 (-4.1656, 29.6037) -> (-4.1656, 41.6687)
  line L21 (-4.1656, 29.6037) -> (-7.112, 29.6037)
  line L22 (-7.112, 29.6037) -> (-7.112, 29.6672)
  line L23 (-14.1224, 29.6672) -> (-7.112, 29.6672)
  line L24 (-14.1224, 10.414) -> (-14.1224, 29.6672)
  line L25 (-3.3909, 10.414) -> (-14.1224, 10.414)
  arc A5 (-3.3274, 10.3505) -> (-3.3909, 10.414) centre (-3.3909, 10.3505) ccw
  line L26 (33.5026, -1.1938) -> (33.5026, 1.2556)
  line L27 (17.8054, -1.1938) -> (33.5026, -1.1938)
  line L28 (17.8054, 1.2556) -> (17.8054, -1.1938)
  line L29 (33.5026, 1.2556) -> (17.8054, 1.2556)
  line L30 (7.1374, 47.1424) -> (27.8892, 47.1424)
  line L31 (7.1374, 49.6062) -> (7.1374, 47.1424)
  line L32 (27.8892, 49.6062) -> (7.1374, 49.6062)
  line L33 (27.8892, 47.1424) -> (27.8892, 49.6062)
  line L34 (58.3946, 1.27) -> (58.3946, -1.1938)
  line L35 (79.2226, 1.27) -> (58.3946, 1.27)
  line L36 (79.2226, -1.1938) -> (79.2226, 1.27)
  line L37 (58.3946, -1.1938) -> (79.2226, -1.1938)
  line L38 (83.4136, 3.3782) -> (83.4136, 49.657)
  line L39 (78.4352, 3.3782) -> (83.4136, 3.3782)
  line L40 (78.4352, 49.657) -> (78.4352, 3.3782)
  line L41 (83.4136, 49.657) -> (78.4352, 49.657)
  line L42 (52.6034, 49.6062) -> (52.6034, 47.1424)
  line L43 (73.3552, 49.6062) -> (52.6034, 49.6062)
  line L44 (73.3552, 47.1424) -> (73.3552, 49.6062)
  line L45 (52.6034, 47.1424) -> (73.3552, 47.1424)
  line L46 (29.8704, 47.1424) -> (50.6222, 47.1424)
  line L47 (29.8704, 49.6062) -> (29.8704, 47.1424)
  line L48 (50.6222, 49.6062) -> (29.8704, 49.6062)
  line L49 (50.6222, 47.1424) -> (50.6222, 49.6062)
  line L50 (35.6616, -1.1938) -> (56.4896, -1.1938)
  line L51 (35.6616, 1.27) -> (35.6616, -1.1938)
  line L52 (56.4896, 1.27) -> (35.6616, 1.27)
  line L53 (56.4896, -1.1938) -> (56.4896, 1.27)
  line L54 (12.3467, 23.0022) -> (12.3467, 21.5941)
  line L55 (15.1117, 23.0022) -> (12.3467, 23.0022)
  line L56 (15.1117, 21.5941) -> (15.1117, 23.0022)
  line L57 (12.3467, 21.5941) -> (15.1117, 21.5941)
  line L58 (-7.2627, 18.1267) -> (-7.2627, 11.634)
  line L59 (-3.9937, 18.1267) -> (-7.2627, 18.1267)
  line L60 (-3.9937, 11.634) -> (-3.9937, 18.1267)
  line L61 (-7.2627, 11.634) -> (-3.9937, 11.634)
  line L62 (2.8777, 19.9119) -> (2.8777, 17.0508)
  line L63 (5.6982, 19.9119) -> (2.8777, 19.9119)
  line L64 (5.6982, 17.0508) -> (5.6982, 19.9119)
  line L65 (2.8777, 17.0508) -> (5.6982, 17.0508)
  line L66 (6.6317, 14.6767) -> (6.6317, 13.9462)
  line L67 (8.2279, 14.6767) -> (6.6317, 14.6767)
  line L68 (8.2279, 13.9462) -> (8.2279, 14.6767)
  line L69 (6.6317, 13.9462) -> (8.2279, 13.9462)
  line L70 (-11.4396, 26.1143) -> (-11.4396, 21.5941)
  line L71 (-8.2765, 26.1143) -> (-11.4396, 26.1143)
  line L72 (-8.2765, 21.5941) -> (-8.2765, 26.1143)
  line L73 (-11.4396, 21.5941) -> (-8.2765, 21.5941)
  line L74 (23.7979, 4.6422) -> (23.7979, 3.9161)
  line L75 (25.3456, 4.6422) -> (23.7979, 4.6422)
  line L76 (25.3456, 3.9161) -> (25.3456, 4.6422)
  line L77 (23.7979, 3.9161) -> (25.3456, 3.9161)
  line L78 (25.9674, 12.5506) -> (25.9674, 11.0937)
  line L79 (26.969, 12.5506) -> (25.9674, 12.5506)
  line L80 (26.969, 11.0937) -> (26.969, 12.5506)
  line L81 (25.9674, 11.0937) -> (26.969, 11.0937)
  line L82 (20.5866, 13.4064) -> (20.5866, 10.1468)
  line L83 (22.4384, 13.4064) -> (20.5866, 13.4064)
  line L84 (22.4384, 10.1468) -> (22.4384, 13.4064)
  line L85 (20.5866, 10.1468) -> (22.4384, 10.1468)
  line L86 (13.1069, 19.0982) -> (13.1069, 18.337)
  line L87 (14.6707, 19.0982) -> (13.1069, 19.0982)
  line L88 (14.6707, 18.337) -> (14.6707, 19.0982)
  line L89 (13.1069, 18.337) -> (14.6707, 18.337)
  line L90 (-2.8376, 26.8483) -> (-2.8376, 26.1143)
  line L91 (-1.3678, 26.8483) -> (-2.8376, 26.8483)
  line L92 (-1.3678, 26.1143) -> (-1.3678, 26.8483)
  line L93 (-2.8376, 26.1143) -> (-1.3678, 26.1143)
  line L94 (3.5053, 26.9808) -> (3.5053, 26.1143)
  line L95 (5.0811, 26.9808) -> (3.5053, 26.9808)
  line L96 (5.0811, 26.1143) -> (5.0811, 26.9808)
  line L97 (3.5053, 26.1143) -> (5.0811, 26.1143)
  line L98 (9.7366, 26.9808) -> (9.7366, 26.1143)
  line L99 (11.3, 26.9808) -> (9.7366, 26.9808)
  line L100 (11.3, 26.1143) -> (11.3, 26.9808)
  line L101 (9.7366, 26.1143) -> (11.3, 26.1143)
  line L102 (12.7922, 32.175) -> (12.7922, 30.9022)
  line L103 (14.5702, 32.175) -> (12.7922, 32.175)
  line L104 (14.5702, 30.9022) -> (14.5702, 32.175)
  line L105 (12.7922, 30.9022) -> (14.5702, 30.9022)
  line L106 (13.3079, 38.2648) -> (13.3079, 35.0088)
  line L107 (14.1615, 38.2648) -> (13.3079, 38.2648)
  line L108 (14.1615, 35.0088) -> (14.1615, 38.2648)
  line L109 (13.3079, 35.0088) -> (14.1615, 35.0088)
  line L110 (12.9292, 42.1098) -> (12.9292, 41.3551)
  line L111 (14.3655, 42.1098) -> (12.9292, 42.1098)
  line L112 (14.3655, 41.3551) -> (14.3655, 42.1098)
  line L113 (12.9292, 41.3551) -> (14.3655, 41.3551)
  line L114 (-2.9701, 39.8497) -> (-2.9701, 39.0772)
  line L115 (-1.3678, 39.8497) -> (-2.9701, 39.8497)
  line L116 (-1.3678, 39.0772) -> (-1.3678, 39.8497)
  line L117 (-2.9701, 39.0772) -> (-1.3678, 39.0772)
  line L118 (-2.6721, 35.9046) -> (-2.6721, 32.7312)
  line L119 (-1.7091, 35.9046) -> (-2.6721, 35.9046)
  line L120 (-1.7091, 32.7312) -> (-1.7091, 35.9046)
  line L121 (-2.6721, 32.7312) -> (-1.7091, 32.7312)
  line L122 (61.5532, 35.0088) -> (61.5532, 33.5887)
  line L123 (63.3578, 35.0088) -> (61.5532, 35.0088)
  line L124 (63.3578, 33.5887) -> (63.3578, 35.0088)
  line L125 (61.5532, 33.5887) -> (63.3578, 33.5887)
  line L126 (-2.3, 45.1616) -> (-2.3, 41.9097)
  line L127 (-0.4798, 45.1616) -> (-2.3, 45.1616)
  line L128 (-0.4798, 41.9097) -> (-0.4798, 45.1616)
  line L129 (-2.3, 41.9097) -> (-0.4798, 41.9097)
  arc A6 (0.3948, 25.0132) -> (0.3948, 21.2543) centre (0.717, 23.1338) ccw
  line L130 (8.2935, 25.0132) -> (0.3948, 25.0132)
  arc A7 (8.2935, 21.2543) -> (8.2935, 25.0132) centre (7.9713, 23.1338) ccw
  line L131 (0.3948, 21.2543) -> (8.2935, 21.2543)
  circle A8 centre (11.0964, 6.0607) radius 3.302
  line L132 (53.7966, 24.6667) -> (53.7966, 25.3313)
  line L133 (52.7806, 23.6507) -> (53.7966, 24.6667)
  line L134 (49.402, 23.6507) -> (52.7806, 23.6507)
  line L135 (48.386, 24.6667) -> (49.402, 23.6507)
  line L136 (48.386, 25.3313) -> (48.386, 24.6667)
  line L137 (49.402, 26.3473) -> (48.386, 25.3313)
  line L138 (52.7806, 26.3473) -> (49.402, 26.3473)
  line L139 (53.7966, 25.3313) -> (52.7806, 26.3473)
  line L140 (1.7827, 46.235) -> (1.1223, 46.235)
  line L141 (2.7987, 45.219) -> (1.7827, 46.235)
  line L142 (2.7987, 41.8408) -> (2.7987, 45.219)
  line L143 (1.7827, 40.8248) -> (2.7987, 41.8408)
  line L144 (1.1223, 40.8248) -> (1.7827, 40.8248)
  line L145 (0.1063, 41.8408) -> (1.1223, 40.8248)
  line L146 (0.1063, 45.219) -> (0.1063, 41.8408)
  line L147 (1.1223, 46.235) -> (0.1063, 45.219)
  line L148 (6.7103, 46.235) -> (5.6943, 45.219)
  line L149 (7.3707, 46.235) -> (6.7103, 46.235)
  line L150 (8.3867, 45.219) -> (7.3707, 46.235)
  line L151 (8.3867, 41.8408) -> (8.3867, 45.219)
  line L152 (7.3707, 40.8248) -> (8.3867, 41.8408)
  line L153 (6.7103, 40.8248) -> (7.3707, 40.8248)
  line L154 (5.6943, 41.8408) -> (6.7103, 40.8248)
  line L155 (5.6943, 45.219) -> (5.6943, 41.8408)
  circle A9 centre (0, 48.3362) radius 1.5621
  circle A10 centre (0, 0) radius 1.5621
  circle A11 centre (82.6262, 0) radius 1.5621
  circle A12 centre (51.6255, 4.8785) radius 1.5621
  circle A13 centre (51.6255, 32.8947) radius 1.3153
  circle A14 centre (75.1332, 48.3362) radius 1.5621
  line L156 (3.9163, 46.235) -> (2.9003, 45.219)
  line L157 (4.5767, 46.235) -> (3.9163, 46.235)
  line L158 (5.5927, 45.219) -> (4.5767, 46.235)
  line L159 (5.5927, 41.8408) -> (5.5927, 45.219)
  line L160 (4.5767, 40.8248) -> (5.5927, 41.8408)
  line L161 (3.9163, 40.8248) -> (4.5767, 40.8248)
  line L162 (2.9003, 41.8408) -> (3.9163, 40.8248)
  line L163 (2.9003, 45.219) -> (2.9003, 41.8408)
  line L164 (53.7966, 21.8727) -> (53.7966, 22.5373)
  line L165 (52.7806, 20.8567) -> (53.7966, 21.8727)
  line L166 (49.402, 20.8567) -> (52.7806, 20.8567)
  line L167 (48.386, 21.8727) -> (49.402, 20.8567)
  line L168 (48.386, 22.5373) -> (48.386, 21.8727)
  line L169 (49.402, 23.5533) -> (48.386, 22.5373)
  line L170 (52.7806, 23.5533) -> (49.402, 23.5533)
  line L171 (53.7966, 22.5373) -> (52.7806, 23.5533)
  line L172 (53.7966, 27.4607) -> (53.7966, 28.1253)
  line L173 (52.7806, 26.4447) -> (53.7966, 27.4607)
  line L174 (49.402, 26.4447) -> (52.7806, 26.4447)
  line L175 (48.386, 27.4607) -> (49.402, 26.4447)
  line L176 (48.386, 28.1253) -> (48.386, 27.4607)
  line L177 (49.402, 29.1413) -> (48.386, 28.1253)
  line L178 (52.7806, 29.1413) -> (49.402, 29.1413)
  line L179 (53.7966, 28.1253) -> (52.7806, 29.1413)
  circle A15 centre (3.9075, 6.0607) radius 3.302
  line L180 (57.1918, 28.2371) -> (57.1918, 21.9581)
  line L181 (63.6527, 28.2371) -> (57.1918, 28.2371)
  line L182 (63.6527, 21.9581) -> (63.6527, 28.2371)
  line L183 (57.1918, 21.9581) -> (63.6527, 21.9581)
  line L184 (66.3035, 35.9046) -> (66.3035, 32.5006)
  line L185 (67.5508, 35.9046) -> (66.3035, 35.9046)
  line L186 (67.5508, 32.5006) -> (67.5508, 35.9046)
  line L187 (66.3035, 32.5006) -> (67.5508, 32.5006)
  line L188 (-2.9701, 32.0256) -> (-2.9701, 31.0896)
  line L189 (-1.3678, 32.0256) -> (-2.9701, 32.0256)
  line L190 (-1.3678, 31.0896) -> (-1.3678, 32.0256)
  line L191 (-2.9701, 31.0896) -> (-1.3678, 31.0896)
  line L192 (-2.9701, 37.5322) -> (-2.9701, 36.6368)
  line L193 (-1.3678, 37.5322) -> (-2.9701, 37.5322)
  line L194 (-1.3678, 36.6368) -> (-1.3678, 37.5322)
  line L195 (-2.9701, 36.6368) -> (-1.3678, 36.6368)
  line L196 (-6.9964, 42.9992) -> (-6.9964, 41.9097)
  line L197 (-5.0545, 42.9992) -> (-6.9964, 42.9992)
  line L198 (-5.0545, 41.9097) -> (-5.0545, 42.9992)
  line L199 (-6.9964, 41.9097) -> (-5.0545, 41.9097)
  line L200 (12.7922, 40.0541) -> (12.7922, 38.8221)
  line L201 (14.5702, 40.0541) -> (12.7922, 40.0541)
  line L202 (14.5702, 38.8221) -> (14.5702, 40.0541)
  line L203 (12.7922, 38.8221) -> (14.5702, 38.8221)
  line L204 (12.7922, 34.4881) -> (12.7922, 33.2287)
  line L205 (14.5702, 34.4881) -> (12.7922, 34.4881)
  line L206 (14.5702, 33.2287) -> (14.5702, 34.4881)
  line L207 (12.7922, 33.2287) -> (14.5702, 33.2287)
  line L208 (13.3079, 29.9286) -> (13.3079, 26.7098)
  line L209 (14.3655, 29.9286) -> (13.3079, 29.9286)
  line L210 (14.3655, 26.7098) -> (14.3655, 29.9286)
  line L211 (13.3079, 26.7098) -> (14.3655, 26.7098)
  line L212 (6.6317, 26.9808) -> (6.6317, 26.1143)
  line L213 (8.1119, 26.9808) -> (6.6317, 26.9808)
  line L214 (8.1119, 26.1143) -> (8.1119, 26.9808)
  line L215 (6.6317, 26.1143) -> (8.1119, 26.1143)
  line L216 (0.2905, 26.8483) -> (0.2905, 26.1143)
  line L217 (1.8236, 26.8483) -> (0.2905, 26.8483)
  line L218 (1.8236, 26.1143) -> (1.8236, 26.8483)
  line L219 (0.2905, 26.1143) -> (1.8236, 26.1143)
  line L220 (-2.9701, 28.4771) -> (-2.9701, 27.8018)
  line L221 (-1.3678, 28.4771) -> (-2.9701, 28.4771)
  line L222 (-1.3678, 27.8018) -> (-1.3678, 28.4771)
  line L223 (-2.9701, 27.8018) -> (-1.3678, 27.8018)
  line L224 (13.0148, 15.7926) -> (13.0148, 15.0444)
  line L225 (14.5702, 15.7926) -> (13.0148, 15.7926)
  line L226 (14.5702, 15.0444) -> (14.5702, 15.7926)
  line L227 (13.0148, 15.0444) -> (14.5702, 15.0444)
  line L228 (23.6729, 13.4064) -> (23.6729, 10.1468)
  line L229 (24.9476, 13.4064) -> (23.6729, 13.4064)
  line L230 (24.9476, 10.1468) -> (24.9476, 13.4064)
  line L231 (23.6729, 10.1468) -> (24.9476, 10.1468)
  line L232 (18.9382, 13.024) -> (18.9382, 10.8934)
  line L233 (19.9033, 13.024) -> (18.9382, 13.024)
  line L234 (19.9033, 10.8934) -> (19.9033, 13.024)
  line L235 (18.9382, 10.8934) -> (19.9033, 10.8934)
  line L236 (-5.6282, 24.3602) -> (-5.6282, 21.5941)
  line L237 (-4.4808, 24.3602) -> (-5.6282, 24.3602)
  line L238 (-4.4808, 21.5941) -> (-4.4808, 24.3602)
  line L239 (-5.6282, 21.5941) -> (-4.4808, 21.5941)
  line L240 (-0.1051, 15.5086) -> (-0.1051, 13.9462)
  line L241 (0.6862, 15.5086) -> (-0.1051, 15.5086)
  line L242 (0.6862, 13.9462) -> (0.6862, 15.5086)
  line L243 (-0.1051, 13.9462) -> (0.6862, 13.9462)
  line L244 (3.872, 15.2448) -> (3.872, 12.0387)
  line L245 (4.8257, 15.2448) -> (3.872, 15.2448)
  line L246 (4.8257, 12.0387) -> (4.8257, 15.2448)
  line L247 (3.872, 12.0387) -> (4.8257, 12.0387)
  line L248 (5.5046, 1.1225) -> (5.5046, -1.3243)
  line L249 (9.5396, 1.1225) -> (5.5046, 1.1225)
  line L250 (9.5396, -1.3243) -> (9.5396, 1.1225)
  line L251 (5.5046, -1.3243) -> (9.5396, -1.3243)
  line L252 (3.1684, 34.4881) -> (3.1684, 29.563)
  line L253 (8.2279, 34.4881) -> (3.1684, 34.4881)
  line L254 (8.2279, 29.563) -> (8.2279, 34.4881)
  line L255 (3.1684, 29.563) -> (8.2279, 29.563)
  line L256 (29.7171, 32.7312) -> (29.7171, 18.5332)
  line L257 (43.7506, 32.7312) -> (29.7171, 32.7312)
  line L258 (43.7506, 18.5332) -> (43.7506, 32.7312)
  line L259 (29.7171, 18.5332) -> (43.7506, 18.5332)
  line L260 (-3.3274, 10.3505) -> (-3.3274, 9.7155)
  arc A16 (-3.3274, 9.7155) -> (-3.2639, 9.652) centre (-3.2639, 9.7155) ccw
  line L261 (-3.2639, 9.652) -> (-1.7907, 9.652)
  arc A17 (-1.7272, 9.5885) -> (-1.7907, 9.652) centre (-1.7907, 9.5885) ccw
  line L262 (-1.7272, 2.0955) -> (-1.7272, 9.5885)
  arc A18 (-1.7907, 2.032) -> (-1.7272, 2.0955) centre (-1.7907, 2.0955) ccw
  line L263 (-1.7907, 2.032) -> (-3.2639, 2.032)
  arc A19 (-3.2639, 2.032) -> (-3.3274, 1.9685) centre (-3.2639, 1.9685) ccw
  line L264 (-3.3274, 1.9685) -> (-3.3274, 1.3335)
  arc A20 (-3.3909, 1.27) -> (-3.3274, 1.3335) centre (-3.3909, 1.3335) ccw
  line L265 (-14.1224, 1.27) -> (-3.3909, 1.27)
  line L266 (-14.1224, -1.016) -> (-14.1224, 1.27)
  line L267 (-14.1224, -1.016) -> (-12.5984, -2.54)
  line L268 (83.9216, -2.54) -> (-12.5984, -2.54)
  line L269 (83.9216, -2.54) -> (87.4776, 1.016)
  line L270 (87.4776, 35.6362) -> (87.4776, 1.016)
  line L271 (84.9376, 38.1762) -> (87.4776, 35.6362)
  line L272 (84.9376, 49.1128) -> (84.9376, 38.1762)
  line L273 (83.1742, 50.8762) -> (84.9376, 49.1128)
  line L274 (-12.5984, 50.8762) -> (83.1742, 50.8762)
  line L275 (-12.5984, 50.8762) -> (-14.1224, 49.3522)
  line L276 (-14.1224, 41.6052) -> (-14.1224, 49.3522)
  line L277 (-7.112, 41.6052) -> (-14.1224, 41.6052)
  line L278 (-7.112, 41.6687) -> (-7.112, 41.6052)
  line L279 (-4.1656, 41.6687) -> (-7.112, 41.6687)
  line L280 (-4.1656, 29.6037) -> (-4.1656, 41.6687)
  line L281 (-4.1656, 29.6037) -> (-7.112, 29.6037)
  line L282 (-7.112, 29.6037) -> (-7.112, 29.6672)
  line L283 (-14.1224, 29.6672) -> (-7.112, 29.6672)
  line L284 (-14.1224, 10.414) -> (-14.1224, 29.6672)
  line L285 (-3.3909, 10.414) -> (-14.1224, 10.414)
  arc A21 (-3.3274, 10.3505) -> (-3.3909, 10.414) centre (-3.3909, 10.3505) ccw
  line L286 (33.5026, -1.1938) -> (33.5026, 1.2556)
  line L287 (17.8054, -1.1938) -> (33.5026, -1.1938)
  line L288 (17.8054, 1.2556) -> (17.8054, -1.1938)
  line L289 (33.5026, 1.2556) -> (17.8054, 1.2556)
  line L290 (7.1374, 47.1424) -> (27.8892, 47.1424)
  line L291 (7.1374, 49.6062) -> (7.1374, 47.1424)
  line L292 (27.8892, 49.6062) -> (7.1374, 49.6062)
  line L293 (27.8892, 47.1424) -> (27.8892, 49.6062)
  line L294 (58.3946, 1.27) -> (58.3946, -1.1938)
  line L295 (79.2226, 1.27) -> (58.3946, 1.27)
  line L296 (79.2226, -1.1938) -> (79.2226, 1.27)
  line L297 (58.3946, -1.1938) -> (79.2226, -1.1938)
  line L298 (83.4136, 3.3782) -> (83.4136, 49.657)
  line L299 (78.4352, 3.3782) -> (83.4136, 3.3782)
  line L300 (78.4352, 49.657) -> (78.4352, 3.3782)
  line L301 (83.4136, 49.657) -> (78.4352, 49.657)
  line L302 (52.6034, 49.6062) -> (52.6034, 47.1424)
  line L303 (73.3552, 49.6062) -> (52.6034, 49.6062)
  line L304 (73.3552, 47.1424) -> (73.3552, 49.6062)
  line L305 (52.6034, 47.1424) -> (73.3552, 47.1424)
  line L306 (29.8704, 47.1424) -> (50.6222, 47.1424)
  line L307 (29.8704, 49.6062) -> (29.8704, 47.1424)
  line L308 (50.6222, 49.6062) -> (29.8704, 49.6062)
  line L309 (50.6222, 47.1424) -> (50.6222, 49.6062)
  line L310 (35.6616, -1.1938) -> (56.4896, -1.1938)
  line L311 (35.6616, 1.27) -> (35.6616, -1.1938)
  line L312 (56.4896, 1.27) -> (35.6616, 1.27)
  line L313 (56.4896, -1.1938) -> (56.4896, 1.27)
  line L314 (12.3467, 23.0022) -> (12.3467, 21.5941)
  line L315 (15.1117, 23.0022) -> (12.3467, 23.0022)
  line L316 (15.1117, 21.5941) -> (15.1117, 23.0022)